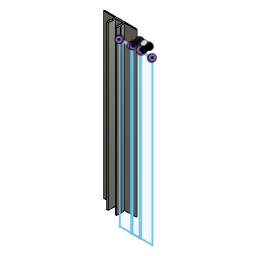
extrusion covers v1 (Autodesk Fusion 360 design; units mm, degrees)
Autodesk Fusion 360 part; units mm, degrees
sketch "cover" plane through (0, 0, 0) normal (0, 0, 1) x (1, 0, 0)
  line L0 (-29.3442, 32.4163) -> (-9.3442, 32.4163)
  line L1 (-9.3442, 32.4163) -> (-9.3442, -67.5837)
  line L2 (-9.3442, -67.5837) -> (-29.3442, -67.5837)
  line L3 (-29.3442, -67.5837) -> (-29.3442, 32.4163)
  line L4 (-22.3942, 32.4163) -> (-16.2942, 32.4163)
  line L5 (-16.2942, 32.4163) -> (-16.2942, -67.5837)
  line L6 (-16.2942, -67.5837) -> (-22.3942, -67.5837)
  line L7 (-22.3942, -67.5837) -> (-22.3942, 32.4163)
  line L8 (-17.1742, -67.5837) -> (-17.1742, 32.4163)
  line L9 (-21.5142, 32.4163) -> (-21.5142, -67.5837)
  dimension "d5" = 20
  dimension "d6" = 100
  dimension "d7" = 6.1
  dimension "d8" = 0.88
  dimension "d9" = 0.88
  constraint horizontal L0
  constraint vertical L1
  constraint horizontal L2
  constraint vertical L3
  constraint horizontal L4
  constraint vertical L5
  constraint horizontal L6
  constraint vertical L7
  constraint midpoint L2 L6
  constraint midpoint L0 L4
  constraint coincident L6 L8.start
  constraint coincident L4 L8.end
  constraint perpendicular L4 L8
  constraint coincident L0 L9.start
  constraint coincident L2 L9.end
  constraint vertical L9
  measures "d5" distance of L0.start L0.end
  measures "d6" distance of L0.start L2.end
  measures "d7" distance of L5 L7
  measures "d8" distance of L5 L8
  measures "d9" distance of L7 L9
extrude "Extrude1" add sketch "cover" along normal blind 0.6
extrude "Extrude2" add sketch "cover" against normal blind 5 contours L0 L2 L4 L6 L7 L9 | L0 L2 L4 L5 L6 L8
extrude "Extrude3" add sketch "cover" against normal blind 0.4 contours L0 L2 L4 L6 L8 L9
sketch "wings" plane through (0, 32.4163, 0) normal (0, 1, 0) x (-1, 0, 0)
  line L0 (22.3942, 0) -> (29.3442, 0)
  line L1 (29.3442, 0) -> (29.3442, 0.6)
  line L2 (29.3442, 0.6) -> (9.3442, 0.6)
  line L3 (9.3442, 0.6) -> (9.3442, 0)
  line L4 (9.3442, 0) -> (16.2942, 0)
  line L5 (16.2942, 0) -> (16.2942, -5)
  line L6 (16.2942, -5) -> (17.1742, -5)
  line L7 (17.1742, -5) -> (17.1742, -0.4)
  line L8 (17.1742, -0.4) -> (21.5142, -0.4)
  line L9 (21.5142, -0.4) -> (21.5142, -5)
  line L10 (21.5142, -5) -> (22.3942, -5)
  line L11 (22.3942, -5) -> (22.3942, 0)
  line L12 (16.2942, -5) -> (15.8942, -2.9983)
  line L13 (15.8942, -2.9983) -> (16.2942, -1.8)
  line L14 (19.3442, 0.6) -> (19.3442, -5) construction
  line L15 (22.3942, -5) -> (22.7942, -2.9983)
  line L16 (22.7942, -2.9983) -> (22.3942, -1.8)
  dimension "d16" = 1.8
  dimension "d17" = 0.4
  constraint coincident L5.end L6.start
  constraint coincident L5 L13.end
  constraint midpoint L2 L14.start
  constraint perpendicular L2 L14
  constraint symmetric L5.end L14 L10.end
  constraint symmetric L12.end L14 L15.end
  constraint symmetric L13.end L14 L16.end
  measures "d16" distance of L4.end L13.end
  measures "d17" distance of L5 L12.end
extrude "Extrude4" add sketch "wings" against normal up to surface (100 mm away) contours L11 L15 L16 | L5 L12 L13
move_body "Move1" bodies 1 to x (-1, 0, 0) y (0, 1, 0) z (0, 0, -1) at (-58.6885, 0, -10)
equation "extrusionLength = 100 mm" comment "the length of the extrusion you want to cover"
equation "extrusionWidth = 20 mm" comment "the width of the extrusion you want to cover (e.g. 20 for 2020)"
equation "coverThickness = 0.6 mm" comment "how thick the outside cover should be"
equation "wingHeight = 5 mm" comment "how far into the extrusion channel the wings go"
equation "d5 = extrusionWidth"
equation "d6 = extrusionLength"
equation "d7 = extrusionSlotWidth"
equation "d8 = wingThickness"
equation "d9 = wingThickness"
equation "d10 = coverThickness"
equation "d12 = -wingHeight"
equation "d16 = lockingMechanismStartDistance"
equation "d17 = lockingMechanismLatchThickness"
equation "extrusionSlotWidth = 6.1 mm" comment "the width of the slot in the extrusion where the wings go"
equation "lockingMechanismLatchThickness = 0.4 mm" comment "see sketch. tweak to ensure proper latching"
equation "lockingMechanismStartDistance = 1.8 mm" comment "see sketch. tweak to ensure proper latching"
equation "wingThickness = 0.88 mm" comment "2 line widths for me makes it bendy but strong enough"
named bodies: "cover"
